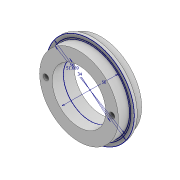
# Autodesk Inventor part: MotorizedRevolver-SM2-adapter
Saved by Autodesk Inventor 2021 (Build 250183000, 183)
## iProperties
Created: 2023-03-14
Part Number: MotorizedRevolver-SM2-adapter
Material: Generic
Document SubType Name: Modeling
Designer: nvladi
Density: 1 g/cm^3
Appearance: Default
Author: nvladi
Autodesk Inventor part; units mm, degrees
ref_plane "YZ Plane" through (0, 0, 0) normal (1, 0, 0) x (0, 1, 0)
ref_plane "XZ Plane" through (0, 0, 0) normal (0, 1, 0) x (-1, 0, 0)
ref_plane "XY Plane" through (0, 0, 0) normal (0, 0, 1) x (1, 0, 0)
sketch "Sketch1" plane through (0, 0, 0) normal (0, 0, 1) x (1, 0, 0)
  circle A0 centre (0, 0) radius 17
  circle A1 centre (0, 0) radius 25.8445
  circle A2 centre (0, 0) radius 28
  circle A3 centre (0, 0) radius 25
  point P0 (-21, 0)
  point P1 (21, 0)
  dimension "d0" = 34
  dimension "d1" = 51.689
  dimension "d2" = 56
  dimension "d3" = 50
  constraints: 4 centre point, 4 coincident
  measures "d0" diameter of A0
  measures "d1" diameter of A1
  measures "d2" diameter of A2
  measures "d3" diameter of A3
extrude "Extrusion1" add sketch "Sketch1" along normal blind 7 contours A3
extrude "Extrusion2" add sketch "Sketch1" against normal blind 2 contours A1 | A2
extrude "Extrusion3" add sketch "Sketch1" against normal blind 7 contours A1 | A3
hole "Hole1" at (-21, 0, 0) at (21, 0, 0) direction (0, 0, -1) diameter 3.5 end through all both
sketch "Sketch2" plane through (0, 0, -7) normal (0, 0, -1) x (-1, 0, 0)
  point P0 (0, 0)
  point P1 (-21, 0)
  point P2 (21, 0)
hole "Hole2" at (-21, 0, -7) at (21, 0, -7) direction (0, 0, 1) diameter 3.5 end through all counterbore diameter 6.5 counterbore depth 4
body "Solid1"
